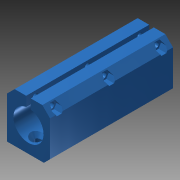
# Autodesk Inventor part: ZAxisCarriageRight
Saved by Autodesk Inventor 2015 SP1 (Build 190203100, 203)
## iProperties
Category: Print
Created: 2014-12-10
Part Number: ZAxisCarriageRight
Material: Generic
Document SubType Name: Modeling
Designer: Jack
Density: 1 g/cm^3
Appearance: Cyan
Mass: 41.893 g
Surface Area: 163.206 cm^2
Volume: 41.893 cm^3
Catalog Web Link: N/A
Author: Jack
Title: Z Axis Carriage Right
Autodesk Inventor part; units mm, degrees
ref_plane "YZ Plane" through (0, 0, 0) normal (1, 0, 0) x (0, 1, 0)
ref_plane "XZ Plane" through (0, 0, 0) normal (0, 1, 0) x (-1, 0, 0)
ref_plane "XY Plane" through (0, 0, 0) normal (0, 0, 1) x (1, 0, 0)
sketch "Sketch1" plane through (0, 0, 0) normal (0, 1, 0) x (-1, 0, 0)
  arc A0 (-1.5, 9.6845) -> (1.5, 9.6845) centre (0, 0) ccw
  line L0 (14, -16) -> (14, 11)
  line L1 (14, 11) -> (9, 16)
  line L2 (9, 16) -> (1.5, 16)
  line L3 (1.5, 16) -> (1.5, 9.6845)
  line L4 (-1.5, 9.6845) -> (-1.5, 16)
  line L5 (-1.5, 16) -> (-9, 16)
  line L6 (-9, 16) -> (-14, 11)
  line L7 (-14, 11) -> (-14, -16)
  line L8 (14, -16) -> (-14, -16)
  dimension "d0" = 19.6
  dimension "d1" = 135
  dimension "d2" = 135
  dimension "d3" = 14
  dimension "d4" = 14
  dimension "d5" = 16
  dimension "d6" = 16
  dimension "d7" = 1.5
  dimension "d8" = 5
  constraints: 18 end point, 2 equal length, 2 parallel, 2 perpendicular, 2 point on circle, 2 point on line, 1 centre point, 1 coincident, 1 horizontal, 1 vertical
  measures "d0" diameter of A0
  measures "d1" angle of L0 L1
  measures "d2" angle of L7 L6
  measures "d3" distance from line of point (0, 0) L0
  measures "d4" distance from line of point (0, 0) L7
  measures "d5" distance from line of point (0, 0) L5
  measures "d6" distance from line of point (0, 0) L8
  measures "d7" distance from line of point (0, 0) L3
  measures "d8" horizontal distance of L6.end L5.end
extrude "Extrusion1" add sketch "Sketch1" along normal blind 80
sketch "Sketch4" plane through (-14, 0, -16) normal (-1, 0, 0) x (0, 0, 1)
  line L0 (0, 0) -> (27, 0) projected
  line L1 (27, 0) -> (27, 80) projected
  line L2 (0, 80) -> (27, 80) projected
  circle A0 centre (28.7, 74) radius 1.75
  circle A1 centre (28.7, 40) radius 1.75
  circle A2 centre (28.7, 6) radius 1.75
  point P0 (-20, 80)
  point P1 (16, 0)
  dimension "d22" = 3.5
  dimension "d23" = 6
  dimension "d24" = 6
  dimension "d25" = 1.7
  dimension "d26" = 40
  constraints: 3 centre point, 2 equal radius, 2 vertical alignment
  measures "d22" diameter of A0
  measures "d23" distance from line of L2 A0.centre
  measures "d24" distance from line of L0 A2.centre
  measures "d25" distance from line of L1 A2.centre
  measures "d26" distance from line of L2 A1.centre
extrude "Extrusion4" cut sketch "Sketch4" against normal up to surface surface through (9, 0, 16) normal (0.7071068, 0, 0.7071068)
sketch "Sketch11" plane through (-14, 0, -16) normal (-1, 0, 0) x (0, 0, 1)
  arc A0 (27, 73.5847) -> (27, 74.4153) centre (28.7, 74) ccw projected
  circle A1 centre (28.7, 74) radius 1.75 projected
  arc A2 (27, 39.5847) -> (27, 40.4153) centre (28.7, 40) ccw projected
  circle A3 centre (28.7, 40) radius 1.75 projected
  arc A4 (27, 5.5847) -> (27, 6.4153) centre (28.7, 6) ccw projected
  circle A5 centre (28.7, 6) radius 1.75 projected
  circle A6 centre (28.7, 74) radius 3.65
  circle A7 centre (28.7, 40) radius 3.65
  circle A8 centre (28.7, 6) radius 3.65
  arc A9 (27, 6.4153) -> (27, 5.5847) centre (28.7, 6) ccw projected
  arc A10 (27, 40.4153) -> (27, 39.5847) centre (28.7, 40) ccw projected
  arc A11 (27, 74.4153) -> (27, 73.5847) centre (28.7, 74) ccw projected
  point P0 (16, 0)
  dimension "d48" = 7.3
  dimension "d49" = 7.3
  dimension "d50" = 7.3
  constraints: 3 centre point, 3 coincident
  measures "d48" diameter of A6
  measures "d49" diameter of A7
  measures "d50" diameter of A8
extrude "Extrusion10" cut sketch "Sketch11" against normal blind 5
sketch "Sketch12" plane through (14, 0, 11) normal (1, 0, 0) x (0, 0, -1)
  circle A0 centre (-1.7, 74) radius 1.75 projected
  arc A1 (0, 74.4153) -> (0, 73.5847) centre (-1.7, 74) ccw projected
  circle A2 centre (-1.7, 40) radius 1.75 projected
  arc A3 (0, 40.4153) -> (0, 39.5847) centre (-1.7, 40) ccw projected
  circle A4 centre (-1.7, 6) radius 1.75 projected
  arc A5 (0, 6.4153) -> (0, 5.5847) centre (-1.7, 6) ccw projected
  line L0 (-4.45, 75.5877) -> (-1.7, 77.1754)
  line L1 (-1.7, 77.1754) -> (1.05, 75.5877)
  line L2 (1.05, 75.5877) -> (1.05, 72.4123)
  line L3 (1.05, 72.4123) -> (-1.7, 70.8246)
  line L4 (-1.7, 70.8246) -> (-4.45, 72.4123)
  line L5 (-4.45, 72.4123) -> (-4.45, 75.5877)
  line L6 (-4.45, 41.5877) -> (-1.7, 43.1754)
  line L7 (-1.7, 43.1754) -> (1.05, 41.5877)
  line L8 (1.05, 41.5877) -> (1.05, 38.4123)
  line L9 (1.05, 38.4123) -> (-1.7, 36.8246)
  line L10 (-1.7, 36.8246) -> (-4.45, 38.4123)
  line L11 (-4.45, 38.4123) -> (-4.45, 41.5877)
  line L12 (-4.45, 7.5877) -> (-1.7, 9.1754)
  line L13 (-1.7, 9.1754) -> (1.05, 7.5877)
  line L14 (1.05, 7.5877) -> (1.05, 4.4123)
  line L15 (1.05, 4.4123) -> (-1.7, 2.8246)
  line L16 (-1.7, 2.8246) -> (-4.45, 4.4123)
  line L17 (-4.45, 4.4123) -> (-4.45, 7.5877)
  arc A6 (0, 5.5847) -> (0, 6.4153) centre (-1.7, 6) ccw projected
  arc A7 (0, 39.5847) -> (0, 40.4153) centre (-1.7, 40) ccw projected
  arc A8 (0, 73.5847) -> (0, 74.4153) centre (-1.7, 74) ccw projected
  point P0 (11, 0)
  point P1 (-1.7, 74)
  point P2 (-1.7, 40)
  point P3 (-1.7, 6)
  dimension "d53" = 5.5
  constraints: 36 end point, 3 coincident, 3 vertical, 2 collinear, 39 other
  measures "d53" distance between parallel lines of L14 L17
extrude "Extrusion11" cut sketch "Sketch12" against normal blind 5
chamfer "Chamfer2" distance 4 angle 45 1 edges at (14, 40, -16)
sketch "Sketch15" plane through (-14, 0, -16) normal (0, 0, -1) x (-1, 0, 0)
  line L0 (-24, 0) -> (0, 0) projected
  line L1 (-24, 80) -> (0, 80) projected
  line L2 (-28, 80) -> (-28, 0) projected
  circle A0 centre (-14, 6) radius 2.25
  circle A1 centre (-14, 40) radius 2.25
  circle A2 centre (-14, 74) radius 2.25
  point P0 (-14, 0)
  dimension "d72" = 4.5
  dimension "d73" = 14
  dimension "d74" = 6
  dimension "d75" = 6
  dimension "d76" = 40
  constraints: 3 centre point, 2 equal radius, 2 vertical alignment
  measures "d72" diameter of A0
  measures "d73" distance from line of L2 A0.centre
  measures "d74" distance from line of L0 A0.centre
  measures "d75" distance from line of L1 A2.centre
  measures "d76" distance from line of A1.centre L1
extrude "Extrusion14" cut sketch "Sketch15" against normal up to next
chamfer "Chamfer3" distance 2.2 angle 45 3 edges at (2.25, 5.9963, -9.5382) (2.25, 39.9963, -9.5382) (2.25, 73.9963, -9.5382)
body "Solid1"
